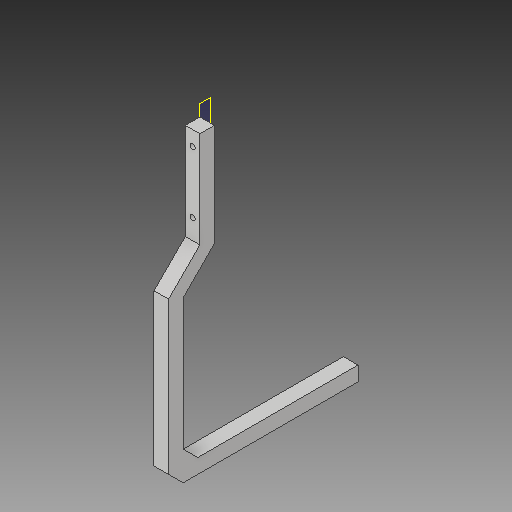
# Autodesk Inventor part: 07_Omnivision_Lamp_arm
Saved by Autodesk Inventor 2019.4 (Build 234330000, 330)
## iProperties
Created: 2021-09-23
Part Number: 07_Omnivision_Lamp_arm
Material: Generisch
Document SubType Name: Modeling
Designer: Muriel
Density: 1 g/cm^3
Appearance: Vorgabe
Author: Muriel
Autodesk Inventor part; units mm, degrees
ref_plane "YZ Plane" through (0, 0, 0) normal (1, 0, 0) x (0, 1, 0)
ref_plane "XZ Plane" through (0, 0, 0) normal (0, 1, 0) x (-1, 0, 0)
ref_plane "XY Plane" through (0, 0, 0) normal (0, 0, 1) x (1, 0, 0)
ref_plane "Arbeitsebene1" through (107, -8, 0) normal (-1, 0, 0) x (0, 0, 1)
sketch "Skizze1" plane through (107, -8, 0) normal (-1, 0, 0) x (0, 0, 1)
  line L0 (-4.1, -2) -> (-4.1, -37.1) projected
  line L1 (0, -2) -> (-4.1, -2) projected
  line L2 (0, -37.1) -> (0, -2) projected
  line L3 (0, -37.1) -> (-4.1, -37.1) projected
  line L4 (0, -37.1) -> (10.7454, -47.8454)
  line L5 (0, -37.1) -> (15.1963, -37.1) construction
  line L6 (10.7454, -47.8454) -> (10.7454, -97.8454)
  line L7 (10.7454, -97.8454) -> (-49.2546, -97.8454)
  line L8 (-49.2546, -97.8454) -> (-49.2546, -102.8454)
  line L9 (-49.2546, -102.8454) -> (15.7454, -102.8454)
  line L10 (15.7454, -102.8454) -> (15.7454, -45.7743)
  line L11 (15.7454, -45.7743) -> (5, -35.0289)
  line L12 (5, -35.0289) -> (5, -2)
  line L13 (5, -2) -> (0, -2)
  line L14 (0, -37.1) -> (0, -2)
  point P0 (0, 8)
  dimension "d0" = 45
  dimension "d1" = 5
  dimension "d2" = 5
  dimension "d3" = 5
  dimension "d4" = 5
  dimension "d5" = 60
  dimension "d6" = 50
  constraints: 22 end point, 5 perpendicular, 2 parallel, 1 collinear, 1 equal length, 1 horizontal, 1 vertical
  measures "d0" angle of L4 L5
  measures "d1" distance of L7.end L8.end
  measures "d2" distance between parallel lines of L2 L12
  measures "d3" distance between parallel lines of L11 L4
  measures "d4" distance between parallel lines of L10 L6
  measures "d5" distance between parallel lines of L6 L8
  measures "d6" distance from line of L4.end L7
extrude "Extrusion1" add sketch "Skizze1" against normal blind 5 contours L13 L12 L11 L10 L9 L8 L7 L6 L4 L2
sketch "Skizze2" plane through (107, -43.0289, 5) normal (0, 0, 1) x (1, 0, 0)
  line L0 (0, 0) -> (0, 33.0289) projected
  line L1 (0, 0) -> (5, 0) projected
  line L2 (5, 33.0289) -> (5, 0) projected
  line L3 (0, 33.0289) -> (5, 33.0289) projected
  circle A0 centre (2.5, 27.9533) radius 0.9
  circle A1 centre (2.5, 6.9011) radius 0.9
  point P0 (-107, 43.0289)
  dimension "d9" = 1.8
  dimension "d10" = 1.8
  constraints: 2 centre point
  measures "d9" diameter of A0
  measures "d10" diameter of A1
extrude "Extrusion2" cut sketch "Skizze2" against normal through all contours A0 | A1
chamfer "Fase1" distance 5 angle 45 2 edges at (109.5, -110.8454, 15.7454) (109.5, -105.8454, 10.7454)
